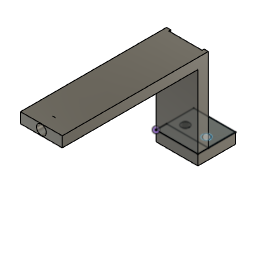
wiperv2 (Autodesk Fusion 360 design; units mm, degrees)
Autodesk Fusion 360 part; units mm, degrees
sketch "Skizze1" plane through (0, 0, 0) normal (0, 0, 1) x (1, 0, 0)
  line L0 (0, 0) -> (20, 0)
  line L1 (20, 0) -> (20, 18)
  line L2 (20, 18) -> (0, 18)
  line L3 (0, 18) -> (0, 0)
  circle A0 centre (15, 9) radius 1.85
  circle A1 centre (5, 9) radius 1.85
  line L4 (0, 0) -> (0, 5)
  line L5 (0, 5) -> (20, 5)
  dimension "d1" = 20
  dimension "d2" = 18
  dimension "d3" = 3.7
  dimension "d4" = 3.7
  dimension "d5" = 5
  constraint horizontal L0
  constraint vertical L1
  constraint horizontal L2
  constraint vertical L3
  constraint coincident L0.start L3.end
  constraint perpendicular L0 L4
  constraint coincident L1 L5.end
  constraint perpendicular L1 L5
  measures "d1" distance of L0.start L0.end
  measures "d2" distance of L0.start L2.end
  measures "d3" diameter of A0
  measures "d4" diameter of A1
  measures "d5" distance of L0.start L4.end
extrude "Extrusion1" add sketch "Skizze1" along normal blind 40 contours L0 L1 L3 L4 L5
extrude "Extrusion2" add sketch "Skizze1" along normal blind 5 contours L1 L2 L3 L5
box "Grundkörper Quader1" add length 5 width 20 height 65 placed x (0, 0, -1) y (1, 0, 0) z (0, -1, 0) at (0, 0, 40)
box "Grundkörper Quader2" cut length 1 width 10 height -35 placed x (0, 0, -1) y (1, 0, 0) z (0, -1, 0) at (5, 0, 35)
extrude "Extrusion3" cut 1 faces at (15, 3.3333, 34.3333) along direction (1, 0, 0) blind 3
extrude "Extrusion4" cut 1 faces at (5, 3.3333, 34.3333) along direction (-1, 0, 0) blind 3
box "Grundkörper Quader3" cut length 5 width 16 height -1 placed x (0, 0, 1) y (1, 0, 0) z (0, 1, 0) at (2, 5, 35)
hole "Bohrung1" at (10, -65, 37.5) direction (0, 1, 0) diameter 4.75 depth 6 tip angle 180
extrude "Extrusion5" add sketch "Skizze1" against normal blind 5
extrude "Extrusion6" cut 1 faces at (8.5586, 15.574, 5) along direction (0, 0, -1) blind 5
